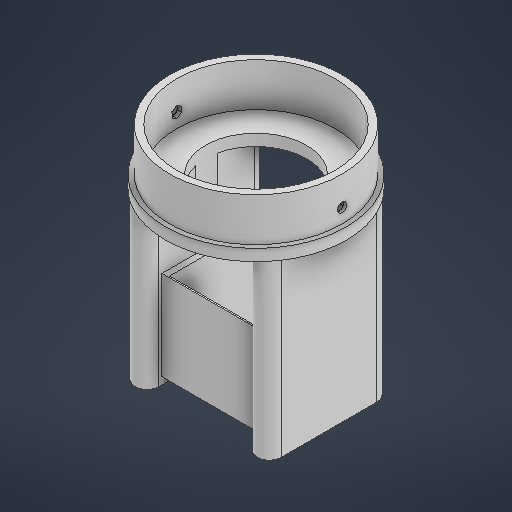
# Autodesk Inventor part: cam_mount90
Saved by Autodesk Inventor 2027 (Build 310192060, 192F)
## iProperties
Created: 2026-07-16
Part Number: cam_mount90
Material: Generic
Document SubType Name: Modeling
Designer: farde
Density: 1 g/cm^3
Appearance: Default
Author: farde
Autodesk Inventor part; units mm, degrees
ref_plane "YZ Plane" through (0, 0, 0) normal (1, 0, 0) x (0, 1, 0)
ref_plane "XZ Plane" through (0, 0, 0) normal (0, 1, 0) x (-1, 0, 0)
ref_plane "XY Plane" through (0, 0, 0) normal (0, 0, 1) x (1, 0, 0)
sketch "Sketch1" plane through (0, 0, 0) normal (0, 1, 0) x (-1, 0, 0)
  circle A0 centre (0, 0) radius 29.85
  circle A1 centre (0, 0) radius 27.5
  dimension "d0" = 59.7
  dimension "d1" = 55
  constraints: 2 centre point, 2 coincident
  measures "d0" diameter of A0
  measures "d1" diameter of A1
extrude "Extrusion1" add sketch "Sketch1" along normal blind 15
sketch "Sketch2" plane through (0, 0, 0) normal (0, 1, 0) x (-1, 0, 0)
  circle A0 centre (0, 0) radius 31.4135
  circle A1 centre (0, 0) radius 28.9404
  circle A2 centre (0, 0) radius 31.4135
  circle A3 centre (0, 0) radius 20.0919
  dimension "d6" = 40.1837
  constraints: 4 centre point, 4 coincident, 1 concentric
  measures "d6" diameter of A3
extrude "Extrusion2" add sketch "Sketch2" against normal blind 4 contours A0 | A1 | A3
sketch "Sketch3" plane through (0, -4, 0) normal (0, -1, 0) x (1, 0, 0)
  line L0 (21.2066, 16.5968) -> (21.2066, -16.5968) construction
  line L1 (17.0959, 16.5968) -> (17.0959, -16.5968)
  line L2 (25.3174, -16.5968) -> (25.3174, 16.5968)
  arc A0 (25.3174, 16.5968) -> (17.0959, 16.5968) centre (21.2066, 16.5968) ccw
  arc A1 (17.0959, -16.5968) -> (25.3174, -16.5968) centre (21.2066, -16.5968) ccw
  point P0 (0, 0)
  point P1 (21.2066, 0)
  dimension "d28" = 8.2215
  constraints: 8 end point, 4 point on circle, 4 tangent, 2 centre point, 1 midpoint, 1 parallel, 1 vertical
  measures "d28" distance between parallel lines of L1 L2
extrude "Extrusion3" add sketch "Sketch3" along normal blind 60
mirror "Mirror1" about plane through (0, 0, 0) normal (1, 0, 0) of "Extrusion3"
sketch "Sketch4" plane through (0, 0, 0) normal (0, 1, 0) x (1, 0, 0)
  circle A0 centre (0, 0) radius 17.5
  dimension "d11" = 35
  constraints: 1 centre point, 1 coincident
  measures "d11" diameter of A0
extrude "Extrusion4" cut sketch "Sketch4" against normal blind 60
sketch "Sketch5" plane through (17.0959, -64, -16.5968) normal (-1, 0, 0) x (0, 0, 1)
  line L0 (32.0968, 2.4749) -> (1.0968, 2.4749)
  line L1 (1.0968, 2.4749) -> (1.0968, 33.4749)
  line L2 (1.0968, 33.4749) -> (32.0968, 33.4749)
  line L3 (32.0968, 33.4749) -> (32.0968, 2.4749)
  line L4 (32.0968, 2.4749) -> (1.0968, 33.4749) construction
  line L5 (1.0968, 2.4749) -> (32.0968, 33.4749) construction
  point P0 (16.5968, 64)
  point P1 (16.5968, 17.9749)
  dimension "d12" = 31
  dimension "d13" = 31
  constraints: 12 end point, 2 midpoint, 2 parallel, 1 horizontal, 1 perpendicular
  measures "d12" distance of L1.end L2.end
  measures "d13" distance of L0.end L1.end
extrude "Extrusion5" add sketch "Sketch5" along normal blind 36.1875
sketch "Sketch6" plane through (17.0959, -61.5251, -15.5) normal (0, -1, 0) x (1, 0, 0)
  point P0 (-17.0959, 15.5)
sketch "Sketch7" plane through (17.0959, -61.5251, -15.5) normal (0, -1, 0) x (1, 0, 0)
  line L0 (-32.0959, 30.5) -> (-2.0959, 30.5)
  line L1 (-2.0959, 30.5) -> (-2.0959, 0.5)
  line L2 (-2.0959, 0.5) -> (-32.0959, 0.5)
  line L3 (-32.0959, 0.5) -> (-32.0959, 30.5)
  line L4 (-32.0959, 30.5) -> (-2.0959, 0.5) construction
  line L5 (-2.0959, 30.5) -> (-32.0959, 0.5) construction
  point P0 (-17.0959, 15.5)
  dimension "d16" = 30
  dimension "d17" = 30
  constraints: 12 end point, 2 midpoint, 2 parallel, 1 horizontal, 1 perpendicular
  measures "d16" distance of L1.end L2.end
  measures "d17" distance of L0.end L1.end
extrude "Extrusion6" cut sketch "Sketch7" against normal blind 33.0125
sketch "Sketch8" plane through (-25.3174, -64, -16.5968) normal (-1, 0, 0) x (0, 0, 1)
  line L0 (27.33, 20.5912) -> (-74.1146, 20.5912) construction
  line L1 (-74.1146, 20.5912) -> (-74.1146, 156.4096) construction
  line L2 (-74.1146, 156.4096) -> (27.33, 156.4096) construction
  line L3 (27.33, 156.4096) -> (27.33, 20.5912) construction
  spline S0 degree 2 poles (26.738, 25.0947) (26.738, 24.0904) (26.0826, 22.4201) (25.5117, 21.8175) knots 0 0 0 1 2 2 2
  spline S1 degree 2 poles (25.5117, 21.8175) (24.9726, 21.2361) (23.3974, 20.5912) (22.5939, 20.5912) knots 0 0 0 1 2 2 2
  spline S2 degree 2 poles (22.5939, 20.5912) (21.6953, 20.5912) (20.2364, 21.1938) (19.6973, 21.7647) knots 0 0 0 1 2 2 2
  spline S3 degree 2 poles (19.6973, 21.7647) (19.0207, 22.4835) (18.2807, 24.8093) (18.2807, 26.5959) knots 0 0 0 1 2 2 2
  spline S4 degree 2 poles (18.2807, 26.5959) (18.2807, 28.2134) (19.0101, 31.11) (19.7184, 32.072) knots 0 0 0 1 2 2 2
  spline S5 degree 2 poles (19.7184, 32.072) (20.469, 33.0869) (22.5834, 34.1547) (24.1268, 34.1547) knots 0 0 0 1 2 2 2
  spline S6 degree 2 poles (24.1268, 34.1547) (24.4757, 34.1547) (25.2686, 34.0807) (25.6069, 33.9749) knots 0 0 0 1 2 2 2
  line L4 (25.6069, 33.9749) -> (25.6069, 32.294)
  line L5 (25.6069, 32.294) -> (25.5223, 32.294)
  spline S7 degree 2 poles (25.5223, 32.294) (25.3003, 32.4209) (24.37, 32.6429) (23.8942, 32.6429) knots 0 0 0 1 2 2 2
  spline S8 degree 2 poles (23.8942, 32.6429) (22.1816, 32.6429) (20.2259, 30.3806) (20.0884, 28.2874) knots 0 0 0 1 2 2 2
  spline S9 degree 2 poles (20.0884, 28.2874) (20.7862, 28.7631) (22.0548, 29.1965) (22.8054, 29.1965) knots 0 0 0 1 2 2 2
  spline S10 degree 2 poles (22.8054, 29.1965) (23.5242, 29.1965) (24.7188, 28.8794) (25.3214, 28.4248) knots 0 0 0 1 2 2 2
  spline S11 degree 2 poles (25.3214, 28.4248) (26.0191, 27.8857) (26.738, 26.247) (26.738, 25.0947) knots 0 0 0 1 2 2 2
  spline S12 degree 2 poles (20.0462, 26.2048) (20.0462, 24.8833) (20.5325, 23.213) (20.9659, 22.7584) knots 0 0 0 1 2 2 2
  spline S13 degree 2 poles (20.9659, 22.7584) (21.3465, 22.3355) (22.1393, 22.0184) (22.6045, 22.0184) knots 0 0 0 1 2 2 2
  spline S14 degree 2 poles (22.6045, 22.0184) (23.6828, 22.0184) (24.962, 23.5618) (24.962, 25.0207) knots 0 0 0 1 2 2 2
  spline S15 degree 2 poles (24.962, 25.0207) (24.962, 25.8453) (24.5391, 26.9131) (24.074, 27.2936) knots 0 0 0 1 2 2 2
  spline S16 degree 2 poles (24.074, 27.2936) (23.7357, 27.5685) (22.9005, 27.7482) (22.4142, 27.7482) knots 0 0 0 1 2 2 2
  spline S17 degree 2 poles (22.4142, 27.7482) (21.8539, 27.7482) (20.5642, 27.3571) (20.0779, 27.0293) knots 0 0 0 1 2 2 2
  spline S18 degree 2 poles (20.0779, 27.0293) (20.0673, 26.9025) (20.0462, 26.469) (20.0462, 26.2048) knots 0 0 0 1 2 2 2
  spline S19 degree 2 poles (8.4702, 27.3782) (8.4702, 30.888) (10.5105, 34.1758) (12.6354, 34.1758) knots 0 0 0 1 2 2 2
  spline S20 degree 2 poles (12.6354, 34.1758) (14.792, 34.1758) (16.8112, 30.8246) (16.8112, 27.3888) knots 0 0 0 1 2 2 2
  spline S21 degree 2 poles (16.8112, 27.3888) (16.8112, 23.8578) (14.7709, 20.5912) (12.6354, 20.5912) knots 0 0 0 1 2 2 2
  spline S22 degree 2 poles (12.6354, 20.5912) (10.4894, 20.5912) (8.4702, 23.9741) (8.4702, 27.3782) knots 0 0 0 1 2 2 2
  spline S23 degree 2 poles (10.7114, 31.3532) (10.4576, 30.7083) (10.2462, 28.7208) (10.2462, 27.3782) knots 0 0 0 1 2 2 2
  spline S24 degree 2 poles (10.2462, 27.3782) (10.2462, 26.0356) (10.4576, 24.0587) (10.7219, 23.3927) knots 0 0 0 1 2 2 2
  spline S25 degree 2 poles (10.7219, 23.3927) (10.9862, 22.7267) (11.906, 22.0395) (12.6354, 22.0395) knots 0 0 0 1 2 2 2
  spline S26 degree 2 poles (12.6354, 22.0395) (13.3649, 22.0395) (14.3057, 22.7267) (14.5806, 23.4138) knots 0 0 0 1 2 2 2
  spline S27 degree 2 poles (14.5806, 23.4138) (14.8449, 24.0799) (15.0352, 26.1096) (15.0352, 27.3888) knots 0 0 0 1 2 2 2
  spline S28 degree 2 poles (15.0352, 27.3888) (15.0352, 28.7631) (14.866, 30.6026) (14.5912, 31.3214) knots 0 0 0 1 2 2 2
  spline S29 degree 2 poles (14.5912, 31.3214) (14.3375, 31.998) (13.3966, 32.7275) (12.6354, 32.7275) knots 0 0 0 1 2 2 2
  spline S30 degree 2 poles (12.6354, 32.7275) (11.9165, 32.7275) (10.9757, 32.0403) (10.7114, 31.3532) knots 0 0 0 1 2 2 2
  spline S31 degree 2 poles (0.1926, 23.9636) (0.1926, 25.3696) (2.1166, 27.2936) (3.5226, 27.2936) knots 0 0 0 1 2 2 2
  spline S32 degree 2 poles (3.5226, 27.2936) (4.9181, 27.2936) (6.8633, 25.3802) (6.8633, 23.9636) knots 0 0 0 1 2 2 2
  spline S33 degree 2 poles (6.8633, 23.9636) (6.8633, 22.5575) (4.9392, 20.6335) (3.5226, 20.6335) knots 0 0 0 1 2 2 2
  spline S34 degree 2 poles (3.5226, 20.6335) (2.1166, 20.6335) (0.1926, 22.5575) (0.1926, 23.9636) knots 0 0 0 1 2 2 2
  spline S35 degree 2 poles (1.5669, 23.9636) (1.5669, 23.1178) (2.6875, 21.9655) (3.5226, 21.9655) knots 0 0 0 1 2 2 2
  spline S36 degree 2 poles (3.5226, 21.9655) (4.3684, 21.9655) (5.489, 23.1178) (5.489, 23.9636) knots 0 0 0 1 2 2 2
  spline S37 degree 2 poles (5.489, 23.9636) (5.489, 24.8199) (4.3472, 25.9616) (3.5226, 25.9616) knots 0 0 0 1 2 2 2
  spline S38 degree 2 poles (3.5226, 25.9616) (2.6875, 25.9616) (1.5669, 24.7987) (1.5669, 23.9636) knots 0 0 0 1 2 2 2
  point P0 (16.5968, 64)
  constraints: 2 other
extrude "Extrusion7" cut sketch "Sketch8" against normal blind 2
sketch "Sketch9" plane through (0, 0, 0) normal (1, 0, 0) x (0, 1, 0)
  circle A0 centre (5, 0) radius 1.6
  line L0 (0, -31.4135) -> (0, 31.4135) projected
  point P0 (0, 0)
  dimension "d22" = 3.2
  dimension "d25" = 5
  constraints: 1 centre point
  measures "d22" diameter of A0
  measures "d25" distance from line of L0 A0.centre
extrude "Extrusion8" cut sketch "Sketch9" along normal mid plane 78.2
sketch "Sketch10" plane through (0, 0, 0) normal (1, 0, 0) x (0, 1, 0)
  line L0 (5.9683, -1.6274) -> (4.0574, -1.6823)
  line L1 (4.0574, -1.6823) -> (3.0544, -0.0549)
  line L2 (3.0544, -0.0549) -> (3.9623, 1.6274)
  line L3 (3.9623, 1.6274) -> (5.8731, 1.6823)
  line L4 (5.8731, 1.6823) -> (6.8761, 0.0549)
  line L5 (6.8761, 0.0549) -> (5.9683, -1.6274)
  point P0 (0, 0)
  point P1 (4.9653, 0)
  constraints: 12 end point, 13 other
extrude "Extrusion9" cut sketch "Sketch10" along normal mid plane 57.5625
body "Solid1"
